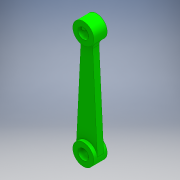
# Autodesk Inventor part: Biella
Saved by Autodesk Inventor 2016 (Build 200138000, 138)
## iProperties
Created: 2016-09-10
Part Number: Biella
Material: Generic
Document SubType Name: Modeling
Designer: Muhammad
Density: 1 g/cm^3
Appearance: Default
Author: Muhammad
Autodesk Inventor part; units mm, degrees
ref_plane "YZ Plane" through (0, 0, 0) normal (1, 0, 0) x (0, 1, 0)
ref_plane "XY Plane" through (0, 0, 0) normal (0, 0, 1) x (1, 0, 0)
sketch "Sketch1" plane through (0, 0, 0) normal (0, 1, 0) x (-1, 0, 0)
  circle A0 centre (0, 0) radius 5
  circle A1 centre (0, 0) radius 2.5
  dimension "d0" = 10
  dimension "d1" = 5
  constraints: 2 centre point, 2 coincident
  measures "d0" diameter of A0
  measures "d1" diameter of A1
extrude "Extrusion1" add sketch "Sketch1" along normal mid plane 6.35
sketch "Sketch2" plane through (0, 0, 0) normal (0, 1, 0) x (-1, 0, 0)
  circle A0 centre (0, 0) radius 2.5 construction
  line L0 (0, 0) -> (0, -49.8) construction
  circle A1 centre (0, -49.8) radius 5
  circle A2 centre (0, -49.8) radius 2.5
  dimension "d4" = 49.8
  dimension "d5" = 10
  constraints: 2 centre point, 2 coincident, 2 end point, 1 vertical
  measures "d4" distance of L0.start L0.end
  measures "d5" diameter of A1
extrude "Extrusion2" add sketch "Sketch2" along normal mid plane 6.35
sketch "Sketch3" plane through (0, 0, 0) normal (1, 0, 0) x (0, 1, 0)
  point P0 (0, 0)
ref_plane "Work Plane1" through (0, 1.5, 0) normal (0, 1, 0) x (-1, 0, 0)
sketch "Sketch4" plane through (0, 1.5, 0) normal (0, 1, 0) x (-1, 0, 0)
  circle A0 centre (0, 0) radius 2.5 projected
  line L0 (-2.5, 0) -> (-5, -49.8)
  circle A1 centre (0, -49.8) radius 5 projected
  line L1 (2.5, 0) -> (5, -49.8)
  constraints: 4 end point, 4 point on circle
extrude "Extrusion3" add sketch "Sketch4" against normal blind 3 contours L1 A1 L0 A0 | L1 A1 L0
sketch "Sketch5" plane through (0, 1.5, -49.8) normal (0, 1, 0) x (1, 0, 0)
  circle A0 centre (0, 0) radius 2.5
  point P0 (0, -49.8)
  constraints: 1 centre point
extrude "Extrusion4" cut sketch "Sketch5" against normal through all
fillet "Fillet1" radius 3 4 edges at (2.7109, 0.75, -4.2013) (2.7109, -0.75, -4.2013) (-2.7109, 0.75, -4.2013) (-2.7109, -0.75, -4.2013)
sketch "Sketch6" plane through (0, 0, 0) normal (1, 0, 0) x (0, 1, 0)
  circle A0 centre (0, 0) radius 1.5
  dimension "d15" = 3
  constraints: 1 centre point, 1 coincident
  measures "d15" diameter of A0
extrude "Extrusion5" cut sketch "Sketch6" against normal through all
body "Solid1"
